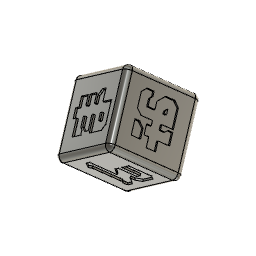
Dice (NKO) v1 (Autodesk Fusion 360 design; units mm, degrees)
Autodesk Fusion 360 part; units mm, degrees
box "直方体プリミティブ1" add length 16 width 16 height 16 placed x (0, -1, 0) y (1, 0, 0) z (0, 0, 1) at (-8, 8, 0)
fillet "フィレット1" radius 1.2 6 faces at (2.6667, 2.6667, 16) (-2.6667, -8, 5.3333) (8, -2.6667, 5.3333) (-2.6667, 8, 5.3333) (-8, -2.6667, 5.3333) (2.6667, 2.6667, 0)
sketch "スケッチ2" plane through (0, -8, 0) normal (0, -1, 0) x (1, 0, 0)
  line L0 (-6.8, 14.8) -> (-6.8, 1.2)
  line L1 (-6.8, 1.2) -> (6.8, 1.2)
  line L2 (6.8, 1.2) -> (6.8, 14.8)
  line L3 (6.8, 14.8) -> (-6.8, 14.8)
  line L4 (-5.05, 6.55) -> (-5.05, 5.55)
  line L5 (-5.05, 5.55) -> (-3.55, 4.05)
  line L6 (-3.55, 4.05) -> (-3.05, 4.55)
  line L7 (-3.05, 4.55) -> (3.45, 4.55)
  line L8 (3.45, 4.55) -> (3.95, 4.05)
  line L9 (3.95, 4.05) -> (4.95, 4.05)
  line L10 (4.95, 4.05) -> (4.95, 5.55)
  line L11 (4.95, 5.55) -> (2.95, 7.55)
  line L12 (2.95, 7.55) -> (3.95, 7.55)
  line L13 (3.95, 7.55) -> (4.95, 8.55)
  line L14 (4.95, 8.55) -> (4.95, 11.55)
  line L15 (4.95, 11.55) -> (3.95, 12.55)
  line L16 (3.95, 12.55) -> (-1.05, 12.55)
  line L17 (-1.05, 12.55) -> (-1.05, 10.55)
  line L18 (-1.05, 10.55) -> (2.95, 10.55)
  line L19 (2.95, 10.55) -> (2.95, 9.55)
  line L20 (-5.05, 6.55) -> (0.95, 6.55)
  line L21 (0.95, 6.55) -> (-1.05, 8.55)
  line L22 (-1.05, 8.55) -> (-1.05, 9.55)
  line L23 (-1.05, 9.55) -> (2.95, 9.55)
  line L24 (6.8, 14.8) -> (-6.8, 14.8)
  line L25 (-6.8, 14.8) -> (-6.8, 1.2)
  line L26 (-6.8, 1.2) -> (6.8, 1.2)
  line L27 (6.8, 1.2) -> (6.8, 14.8)
  constraint perpendicular L5 L6
  constraint perpendicular L4 L7
  constraint perpendicular L6 L8
  constraint parallel L7 L9
  constraint perpendicular L9 L10
  constraint parallel L8 L11
  constraint perpendicular L10 L12
  constraint perpendicular L11 L13
  constraint parallel L10 L14
  constraint perpendicular L13 L15
  constraint perpendicular L16 L17
  constraint perpendicular L17 L18
  constraint perpendicular L18 L19
  constraint perpendicular L4 L20
  constraint perpendicular L13 L21
  constraint parallel L4 L22
  constraint perpendicular L19 L23
extrude "押し出し1" cut sketch "スケッチ2" against normal blind 0.4 contours L4 L5 L6 L7 L8 L9 L10 L11 L12 L13 L14 L15 L16 L17 L18 L19 L20 L21 L22 L23
sketch "スケッチ3" plane through (8, 0, 0) normal (1, 0, 0) x (0, 1, 0)
  line L0 (6.8, 14.8) -> (-6.8, 14.8)
  line L1 (-6.8, 14.8) -> (-6.8, 1.2)
  line L2 (-6.8, 1.2) -> (6.8, 1.2)
  line L3 (6.8, 1.2) -> (6.8, 14.8)
  line L4 (-2.0014, 12.95) -> (3.45, 12.95)
  line L5 (3, 10.45) -> (3.45, 10.45)
  line L6 (-2.0014, 12.95) -> (-2.55, 12.95)
  line L7 (1.95, 10.95) -> (2.55, 10.45)
  line L8 (2.55, 10.45) -> (3, 10.45)
  line L9 (3.45, 10.45) -> (3.45, 12.95)
  line L10 (-3.55, 10.95) -> (-3.55, 11.95)
  line L11 (-2.55, 12.95) -> (-3.55, 11.95)
  line L12 (-4.05, 8.4389) -> (-3.05, 9.45)
  line L13 (-3.05, 9.45) -> (2.9389, 9.45)
  line L14 (2.9389, 9.45) -> (3.95, 8.45)
  line L15 (3.95, 8.45) -> (3.95, 2.95)
  line L16 (-4.05, 8.4389) -> (-4.05, 7.45)
  line L17 (-4.05, 7.45) -> (1.95, 7.45)
  line L18 (1.95, 7.45) -> (1.95, 4.45)
  line L19 (1.95, 4.45) -> (1.45, 3.95)
  line L20 (1.45, 3.95) -> (1.45, 2.95)
  line L21 (1.45, 2.95) -> (3.95, 2.95)
  line L22 (-6.8, 14.8) -> (-6.8, 1.2)
  line L23 (-6.8, 1.2) -> (6.8, 1.2)
  line L24 (6.8, 1.2) -> (6.8, 14.8)
  line L25 (6.8, 14.8) -> (-6.8, 14.8)
  line L26 (1.95, 10.95) -> (-3.55, 10.95)
  constraint parallel L4 L6
  constraint parallel L5 L8
  constraint perpendicular L5 L9
  constraint perpendicular L12 L14
  constraint perpendicular L8 L15
  constraint perpendicular L13 L18
  constraint perpendicular L13 L20
  constraint perpendicular L20 L21
extrude "押し出し2" cut sketch "スケッチ3" against normal blind 0.4 contours L4 L5 L6 L7 L8 L9 L10 L11 L26 | L12 L13 L14 L15 L16 L17 L18 L19 L20 L21
sketch "スケッチ4" plane through (0, 0, 0) normal (0, 0, -1) x (1, 0, 0)
  line L0 (2, -2) -> (2.5, -2)
  line L1 (4, -4) -> (4, -1.5)
  line L2 (4, -1.5) -> (3, -1.5)
  line L3 (3, -1.5) -> (2.5, -2)
  line L4 (4, -4) -> (2, -4)
  line L5 (2, -4) -> (2, -5)
  line L6 (2, -5) -> (0, -5)
  line L7 (0, -5) -> (0, -4)
  line L8 (0, -4) -> (-4, -4)
  line L9 (-4, -4) -> (-4, -2)
  line L10 (0, -2) -> (-2.5, -2)
  line L11 (-2.5, -2) -> (-4, -2)
  line L12 (0, -2) -> (0, -1)
  line L13 (0, -1) -> (-3, -1)
  line L14 (-3, -1) -> (-4, 0)
  line L15 (-4, 0) -> (-4, 4)
  line L16 (-4, 4) -> (-3, 5)
  line L17 (-3, 5) -> (2, 5)
  line L18 (2, 5) -> (2, 4)
  line L19 (1, 3) -> (-2, 3)
  line L20 (-2, 3) -> (-2, 1)
  line L21 (-2, 1) -> (0.5, 1)
  line L22 (2, 1.5) -> (1, 1.5)
  line L23 (1, 1.5) -> (0.5, 1)
  line L24 (2, 4) -> (1, 3)
  line L25 (-6.8, -6.8) -> (6.8, -6.8)
  line L26 (6.8, -6.8) -> (6.8, 6.8)
  line L27 (6.8, 6.8) -> (-6.8, 6.8)
  line L28 (-6.8, 6.8) -> (-6.8, -6.8)
  line L29 (2, -7) -> (2, -6.8)
  line L30 (2, -5) -> (2, -4)
  line L31 (2, -2) -> (2, 1.5)
  line L32 (2, -7) -> (2, -6.8)
  line L33 (2, -5) -> (2, -4)
  constraint perpendicular L0 L29
  constraint perpendicular L0 L1
  constraint perpendicular L1 L2
  constraint perpendicular L1 L4
  constraint perpendicular L4 L5
  constraint perpendicular L1 L6
  constraint perpendicular L6 L7
  constraint perpendicular L7 L8
  constraint perpendicular L8 L9
  constraint perpendicular L9 L10
  constraint perpendicular L9 L11
  constraint perpendicular L4 L12
  constraint perpendicular L12 L13
  constraint perpendicular L11 L15
  constraint perpendicular L15 L17
  constraint perpendicular L17 L18
  constraint perpendicular L18 L19
  constraint perpendicular L19 L20
  constraint perpendicular L20 L21
  constraint perpendicular L19 L32
  constraint perpendicular L22 L32
  constraint coincident L25 L29.end
  constraint collinear L29 L30
  constraint collinear L31 L32
  constraint collinear L32 L33
extrude "押し出し3" cut sketch "スケッチ4" against normal blind 0.4 contours L0 L1 L2 L3 L4 L5 L6 L7 L8 L9 L10 L11 L12 L13 L14 L15 L16 L17 L18 L19 L20 L21 L22 L23 L24 L30 L31 L33
sketch "スケッチ5" plane through (0, 0, 16) normal (0, 0, 1) x (-1, 0, 0)
  line L0 (6.8, 6.8) -> (-6.8, 6.8)
  line L1 (-6.8, 6.8) -> (-6.8, -6.8)
  line L2 (-6.8, -6.8) -> (6.8, -6.8)
  line L3 (6.8, -6.8) -> (6.8, 6.8)
  line L4 (-2.9, -5) -> (-3.9, -4)
  line L5 (-3.9, -4) -> (-3.9, 0)
  line L6 (3.1, 0) -> (4.1, -1)
  line L7 (4.1, -1) -> (4.1, -4)
  line L8 (4.1, -4) -> (3.1, -5)
  line L9 (3.1, -5) -> (2.1, -5)
  line L10 (2.1, -3.5) -> (2.1, -2)
  line L11 (-1.9, -2) -> (-1.9, -3)
  line L12 (-2.9, -5) -> (-0.9, -5)
  line L13 (-0.9, -5) -> (0.6, -3.5)
  line L14 (-1.4, -2.5) -> (-1.9, -3)
  line L15 (-3.9, 1) -> (-3.9, 3)
  line L16 (-1.4, 5) -> (0.6, 5)
  line L17 (2.1, -2) -> (0.6, -2)
  line L18 (-1.4, -2) -> (-1.9, -2)
  line L19 (-1.4, -2) -> (-1.4, -2.5)
  line L20 (-3.9, 0) -> (-1.4, 0)
  line L21 (0.6, 0) -> (3.1, 0)
  line L22 (0.6, -2) -> (0.6, -3.5)
  line L23 (-2.4, 1) -> (-1.4, 1)
  line L24 (0.6, 1) -> (1.6, 1)
  line L25 (-1.4, 5) -> (-1.4, 3)
  line L26 (-1.4, 1) -> (-1.4, 0)
  line L27 (-3.9, 3) -> (-1.4, 3)
  line L28 (0.6, 3) -> (1.6, 3)
  line L29 (0.6, 5) -> (0.6, 3)
  line L30 (0.6, 1) -> (0.6, 0)
  line L31 (-3.9, 1) -> (-3.9, 0.5)
  line L32 (-3.9, 0.5) -> (-2.9, 0.5)
  line L33 (-2.9, 0.5) -> (-2.4, 1)
  line L34 (1.6, 3) -> (1.6, 1)
  line L35 (2.1, 2) -> (3.1, 1)
  line L36 (3.1, 1) -> (4.1, 1)
  line L37 (4.1, 1) -> (4.1, 4)
  line L38 (4.1, 4) -> (2.1, 4)
  line L39 (2.1, 4) -> (2.1, 2)
  line L40 (2.1, -5) -> (1.6, -5)
  line L41 (1.6, -5) -> (1.6, -4)
  line L42 (1.6, -4) -> (2.1, -3.5)
  constraint perpendicular L5 L20
  constraint parallel L4 L6
  constraint perpendicular L7 L20
  constraint perpendicular L6 L8
  constraint perpendicular L7 L9
  constraint perpendicular L9 L10
  constraint perpendicular L10 L17
  constraint perpendicular L11 L17
  constraint parallel L12 L17
  constraint perpendicular L4 L13
  constraint parallel L20 L23
  constraint perpendicular L15 L23
  constraint coincident L17.end L29
  constraint coincident L18.start L25
  constraint collinear L17 L18
  constraint collinear L19 L25
  constraint collinear L20 L21
  constraint collinear L22 L29
  constraint coincident L23.end L25
  constraint coincident L24.start L29
  constraint collinear L23 L24
  constraint collinear L25 L26
  constraint collinear L27 L28
  constraint collinear L29 L30
  constraint perpendicular L23 L31
  constraint perpendicular L31 L32
  constraint perpendicular L36 L37
  constraint perpendicular L37 L38
  constraint perpendicular L38 L39
  constraint perpendicular L10 L40
  constraint perpendicular L40 L41
extrude "押し出し4" cut sketch "スケッチ5" against normal blind 0.4 contours L4 L5 L6 L7 L8 L9 L10 L12 L13 L15 L16 L17 L20 L21 L22 L23 L24 L25 L26 L27 L28 L29 L30 L31 L32 L33 L34 L40 L41 L42 | L35 L36 L37 L38 L39
sketch "スケッチ6" plane through (-8, 0, 0) normal (-1, 0, 0) x (0, -1, 0)
  line L0 (-6.8, 14.8) -> (-6.8, 1.2)
  line L1 (-6.8, 1.2) -> (6.8, 1.2)
  line L2 (6.8, 1.2) -> (6.8, 14.8)
  line L3 (6.8, 14.8) -> (-6.8, 14.8)
  line L4 (0.6, 3) -> (-1.4, 3)
  line L5 (-1.4, 13.5) -> (0.6, 13.5)
  line L6 (0.6, 13.5) -> (3.1, 13.5)
  line L7 (4.1, 12.5) -> (3.1, 13.5)
  line L8 (2.1, 11.5) -> (0.6, 11.5)
  line L9 (2.1, 11) -> (2.1, 11.5)
  line L10 (2.1, 11) -> (0.6, 11)
  line L11 (-1.4, 11) -> (-3.9, 11)
  line L12 (-3.9, 11) -> (-3.9, 10)
  line L13 (-3.9, 10) -> (-2.9, 9)
  line L14 (4.1, 9) -> (4.1, 12.5)
  line L15 (0.6, 11.5) -> (0.6, 11)
  line L16 (-1.4, 11) -> (-1.4, 13.5)
  line L17 (-2.9, 9) -> (-1.4, 9)
  line L18 (0.6, 9) -> (4.1, 9)
  line L19 (-3.4, 8.5) -> (-3.4, 6.5)
  line L20 (4.1, 6) -> (4.1, 4)
  line L21 (-3.4, 4) -> (-3.4, 6)
  line L22 (0.6, 9) -> (0.6, 8.5)
  line L23 (3.6, 8.5) -> (0.6, 8.5)
  line L24 (-1.4, 8.5) -> (-3.4, 8.5)
  line L25 (-1.4, 8.5) -> (-1.4, 9)
  line L26 (-3.4, 6.5) -> (-1.4, 6.5)
  line L27 (0.6, 6.5) -> (2.6, 6.5)
  line L28 (-3.4, 6) -> (-1.4, 6)
  line L29 (0.6, 6) -> (2.6, 6)
  line L30 (0.6, 6.5) -> (0.6, 6)
  line L31 (0.6, 4) -> (0.6, 3)
  line L32 (4.1, 4) -> (0.6, 4)
  line L33 (-1.4, 4) -> (-3.4, 4)
  line L34 (-1.4, 3) -> (-1.4, 4)
  line L35 (-1.4, 6) -> (-1.4, 6.5)
  line L36 (4.1, 6) -> (4.1, 6.5)
  line L37 (4.1, 6.5) -> (3.1, 6.5)
  line L38 (2.6, 6) -> (3.1, 6.5)
  line L39 (2.6, 6.5) -> (3.6, 7.5)
  line L40 (3.6, 7.5) -> (3.6, 8.5)
  constraint perpendicular L4 L34
  constraint perpendicular L5 L34
  constraint perpendicular L4 L15
  constraint perpendicular L6 L15
  constraint perpendicular L8 L15
  constraint perpendicular L8 L9
  constraint perpendicular L10 L15
  constraint coincident L11.start L34
  constraint perpendicular L11 L34
  constraint perpendicular L10 L12
  constraint perpendicular L15 L17
  constraint perpendicular L14 L17
  constraint coincident L18.start L17
  constraint collinear L15 L22
  constraint collinear L16 L34
  constraint collinear L17 L18
  constraint coincident L27.start L26
  constraint collinear L22 L30
  constraint coincident L24.start L34
  constraint collinear L23 L24
  constraint collinear L25 L34
  constraint collinear L26 L27
  constraint coincident L28.end L34
  constraint collinear L28 L29
  constraint collinear L30 L31
  constraint collinear L32 L33
  constraint collinear L34 L35
  constraint perpendicular L29 L36
  constraint perpendicular L36 L37
  constraint perpendicular L27 L40
extrude "押し出し5" cut sketch "スケッチ6" against normal blind 0.4 contours L4 L5 L6 L7 L11 L12 L13 L14 L16 L17 L18 L19 L20 L21 L22 L23 L24 L25 L26 L27 L28 L29 L30 L31 L32 L33 L34 L35 L36 L37 L38 L39 L40
sketch "スケッチ7" plane through (0, 8, 0) normal (0, 1, 0) x (-1, 0, 0)
  line L0 (6.8, 14.8) -> (-6.8, 14.8)
  line L1 (-6.8, 14.8) -> (-6.8, 1.2)
  line L2 (-6.8, 1.2) -> (6.8, 1.2)
  line L3 (6.8, 1.2) -> (6.8, 14.8)
  line L4 (-5, 4) -> (-3, 4)
  line L5 (-3, 4) -> (-3, 10)
  line L6 (-3, 12) -> (-5, 12)
  line L7 (-5, 12) -> (-5, 4)
  line L8 (4, 4) -> (3, 4)
  line L9 (3, 6) -> (3, 12)
  line L10 (3, 12) -> (5, 12)
  line L11 (5, 12) -> (5, 5)
  line L12 (4, 4) -> (5, 5)
  line L13 (3, 4) -> (1, 4)
  line L14 (1, 4) -> (0, 5)
  line L15 (0, 5) -> (0, 6)
  line L16 (0, 6) -> (3, 6)
  line L17 (-3, 12) -> (-2, 12)
  line L18 (-2, 12) -> (-2, 11)
  line L19 (-2, 11) -> (-3, 10)
  constraint horizontal L4
  constraint vertical L5
  constraint horizontal L6
  constraint vertical L7
  constraint horizontal L8
  constraint vertical L9
  constraint horizontal L10
  constraint vertical L11
  constraint perpendicular L9 L13
  constraint perpendicular L13 L15
  constraint perpendicular L9 L16
  constraint perpendicular L5 L17
  constraint perpendicular L17 L18
extrude "押し出し6" cut sketch "スケッチ7" against normal blind 0.4 contours L4 L5 L6 L7 L17 L18 L19 | L8 L9 L10 L11 L12 L13 L14 L15 L16
move_body "移動4" bodies 1 to x (0.707107, 0.707107, 0) y (-0.707107, 0.707107, 0) z (0, 0, 1) at (0, 0, 0)
move_body "移動5" bodies 1 to x (0.707107, 0, -0.707107) y (0, 1, 0) z (0.707107, 0, 0.707107) at (0, 0, 0)
move_body "移動6" bodies 1 to x (1, 0, 0) y (0, 1, 0) z (0, 0, 1) at (-7.5, 0, 7)
move_body "移動7" bodies 1 to x (0.984808, 0, -0.173648) y (0, 1, 0) z (0.173648, 0, 0.984808) at (0, 0, 0)
move_body "移動8" bodies 1 to x (1, 0, 0) y (0, 1, 0) z (0, 0, 1) at (-0.35, 0, 0.2)
named bodies: "D-NKO"
